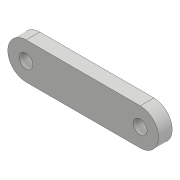
# Autodesk Inventor part: bar2
Saved by Autodesk Inventor 2018 (Build 220112000, 112)
## iProperties
Created: 2018-05-25
Part Number: bar2
Material: Generic
Document SubType Name: Modeling
Designer: Bardo91
Density: 1 g/cm^3
Appearance: Default
Author: Bardo91
Autodesk Inventor part; units mm, degrees
ref_plane "YZ Plane" through (0, 0, 0) normal (1, 0, 0) x (0, 1, 0)
ref_plane "XZ Plane" through (0, 0, 0) normal (0, 1, 0) x (-1, 0, 0)
ref_plane "XY Plane" through (0, 0, 0) normal (0, 0, 1) x (1, 0, 0)
sketch "Sketch1" plane through (0, 0, 0) normal (0, 1, 0) x (-1, 0, 0)
  circle A0 centre (0, 0) radius 1.5
  circle A1 centre (0, 0) radius 4
  line L0 (0, 0) -> (25, 0)
  circle A2 centre (25, 0) radius 4
  circle A3 centre (25, 0) radius 1.5
  line L1 (25, -4) -> (0, -4)
  line L2 (0, 4) -> (25, 4)
  dimension "d0" = 3
  dimension "d1" = 8
  dimension "d4" = 25
  dimension "d5" = 8
  dimension "d6" = 3
  constraints: 6 end point, 4 centre point, 4 coincident, 4 point on circle, 2 horizontal, 2 tangent, 1 parallel
  measures "d0" diameter of A0
  measures "d1" diameter of A1
  measures "d4" distance of L0.start L0.end
  measures "d5" diameter of A2
  measures "d6" diameter of A3
extrude "Extrusion1" add sketch "Sketch1" along normal blind 3
body "Solid1"
